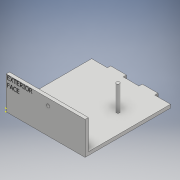
# Autodesk Inventor part: WormGearMount
Saved by Autodesk Inventor 2017 (Build 210142000, 142)
## iProperties
Created: 2016-08-11
Part Number: WormGearMount
Material: Generic
Document SubType Name: Modeling
Designer: Himesh Kurera
Density: 1 g/cm^3
Appearance: Default
Author: Himesh Kurera
Autodesk Inventor part; units mm, degrees
ref_plane "YZ Plane" through (0, 0, 0) normal (1, 0, 0) x (0, 1, 0)
ref_plane "XZ Plane" through (0, 0, 0) normal (0, 1, 0) x (-1, 0, 0)
ref_plane "XY Plane" through (0, 0, 0) normal (0, 0, 1) x (1, 0, 0)
sketch "Sketch1" plane through (0, 0, 0) normal (0, 0, 1) x (1, 0, 0)
  line L0 (0, 0) -> (120, 0)
  line L1 (120, 0) -> (120, 135)
  line L2 (120, 135) -> (0, 135)
  line L3 (0, 135) -> (0, 0)
  dimension "d0" = 120
  dimension "d1" = 135
  constraints: 8 end point, 2 parallel, 1 horizontal, 1 perpendicular
  measures "d0" distance of L2.end L1.end
  measures "d1" distance of L1.end L0.end
extrude "Extrusion1" add sketch "Sketch1" along normal blind 5
sketch "Sketch2" plane through (0, 0, 5) normal (0, 0, 1) x (1, 0, 0)
  line L0 (0, 0) -> (120, 0) projected
  line L1 (0, 0) -> (120, 0)
  line L2 (120, 0) -> (120, 5)
  line L3 (120, 5) -> (0, 5)
  line L4 (0, 5) -> (0, 0)
  dimension "d4" = 120
  dimension "d5" = 5
  constraints: 8 end point, 2 parallel, 1 horizontal, 1 perpendicular
  measures "d4" distance of L3.end L2.end
  measures "d5" distance of L2.end L1.end
extrude "Extrusion2" add sketch "Sketch2" along normal blind 45
sketch "Sketch3" plane through (0, 0, 5) normal (0, 0, 1) x (1, 0, 0)
  line L0 (120, 135) -> (0, 135) projected
  line L1 (0, 135) -> (24, 135)
  line L2 (24, 135) -> (24, 130)
  line L3 (24, 130) -> (0, 130)
  line L4 (0, 130) -> (0, 135)
  line L5 (120, 135) -> (96, 135)
  line L6 (96, 135) -> (96, 130)
  line L7 (96, 130) -> (120, 130)
  line L8 (120, 130) -> (120, 135)
  line L9 (48, 135) -> (72, 135)
  line L10 (72, 135) -> (72, 130)
  line L11 (72, 130) -> (48, 130)
  line L12 (48, 130) -> (48, 135)
  point P0 (0, 0)
  dimension "d8" = 24
  dimension "d9" = 5
  dimension "d10" = 24
  dimension "d11" = 5
  dimension "d12" = 24
  dimension "d13" = 24
  constraints: 24 end point, 6 parallel, 3 horizontal, 3 perpendicular, 2 point on line
  measures "d8" distance of L2.end L3.end
  measures "d9" distance of L1.end L2.end
  measures "d10" distance of L7.end L6.end
  measures "d11" distance of L6.end L5.end
  measures "d12" distance of L10.end L11.end
  measures "d13" distance between parallel lines of L12 L2
extrude "Extrusion3" cut sketch "Sketch3" against normal blind 45
sketch "Sketch4" plane through (0, 0, 5) normal (0, 0, 1) x (1, 0, 0)
  line L0 (1.8933, 18.6085) -> (59.744, 18.6085) construction
  line L1 (59.744, 18.6085) -> (59.744, 5.8096) construction
  line L2 (59.744, 5.8096) -> (1.8933, 5.8096) construction
  line L3 (1.8933, 5.8096) -> (1.8933, 18.6085) construction
  point P0 (0, 0)
  constraints: 2 other
sketch "Sketch5" plane through (0, 0, 0) normal (0, -1, 0) x (1, 0, 0)
  line L0 (1.2536, 49.5181) -> (91.5145, 49.5181) construction
  line L1 (91.5145, 49.5181) -> (91.5145, 35.1014) construction
  line L2 (91.5145, 35.1014) -> (1.2536, 35.1014) construction
  line L3 (1.2536, 35.1014) -> (1.2536, 49.5181) construction
  point P0 (0, 0)
  constraints: 2 other
sketch "Sketch6" plane through (0, 5, 5) normal (0, 1, 0) x (1, 0, 0)
  line L0 (39.1274, -43.5353) -> (-30.0492, -43.5353) construction
  line L1 (-30.0492, -43.5353) -> (-30.0492, -68.4744) construction
  line L2 (-30.0492, -68.4744) -> (39.1274, -68.4744) construction
  line L3 (39.1274, -68.4744) -> (39.1274, -43.5353) construction
  point P0 (0, 5)
  constraints: 2 other
sketch "Sketch7" plane through (0, 0, 0) normal (0, 0, -1) x (-1, 0, 0)
  line L0 (-119.0942, 8.7754) -> (-47.9511, 8.7754) construction
  line L1 (-47.9511, 8.7754) -> (-47.9511, -14.4167) construction
  line L2 (-47.9511, -14.4167) -> (-119.0942, -14.4167) construction
  line L3 (-119.0942, -14.4167) -> (-119.0942, 8.7754) construction
  point P0 (0, 0)
  constraints: 2 other
sketch "Sketch8" plane through (0, 0, 0) normal (0, -1, 0) x (1, 0, 0)
  point P0 (0, 0)
sketch "Sketch9" plane through (0, 0, 0) normal (0, -1, 0) x (1, 0, 0)
  line L0 (120, 0) -> (120, 5) projected
  line L1 (120, 0) -> (120, 39.815)
  line L2 (120, 39.815) -> (64, 39.815)
  circle A0 centre (64, 39.815) radius 2.5
  point P0 (0, 0)
  dimension "d18" = 39.815
  dimension "d19" = 56
  dimension "d20" = 5
  constraints: 4 end point, 1 centre point, 1 coincident, 1 collinear, 1 perpendicular
  measures "d18" distance of L0.start L1.end
  measures "d19" distance of L1.end L2.end
  measures "d20" diameter of A0
extrude "Extrusion4" cut sketch "Sketch9" against normal blind 10
sketch "Sketch10" plane through (0, 0, 5) normal (0, 0, 1) x (1, 0, 0)
  point P0 (0, 0)
sketch "Sketch11" plane through (0, 0, 5) normal (0, 0, 1) x (1, 0, 0)
  line L0 (120, 5) -> (120, 130) projected
  line L1 (120, 5) -> (90, 5)
  line L2 (120, 5) -> (0, 5) projected
  line L3 (90, 5) -> (90, 80)
  circle A0 centre (90, 80) radius 2.5
  point P0 (0, 0)
  dimension "d23" = 30
  dimension "d24" = 75
  dimension "d25" = 5
  constraints: 4 end point, 1 centre point, 1 coincident, 1 perpendicular, 1 point on line
  measures "d23" distance of L0.start L1.end
  measures "d24" distance of L1.end L3.end
  measures "d25" diameter of A0
extrude "Extrusion5" add sketch "Sketch11" along normal blind 38.1
body "Solid1"
